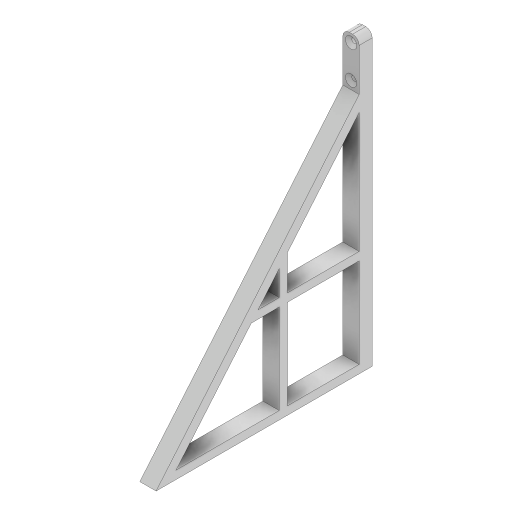
# Autodesk Inventor part: legs
Saved by Autodesk Inventor 2023 (Build 270158000, 158)
## iProperties
Created: 2023-10-18
Part Number: legs
Material: Generic
Document SubType Name: Modeling
Designer: MVeszpremi
Density: 1 g/cm^3
Appearance: Default
Author: MVeszpremi
Autodesk Inventor part; units mm, degrees
ref_plane "YZ Plane" through (0, 0, 0) normal (1, 0, 0) x (0, 1, 0)
ref_plane "XZ Plane" through (0, 0, 0) normal (0, 1, 0) x (-1, 0, 0)
ref_plane "XY Plane" through (0, 0, 0) normal (0, 0, 1) x (1, 0, 0)
sketch "Sketch1" plane through (0, 0, 0) normal (0, 0, 1) x (1, 0, 0)
  line L0 (0, 0) -> (0, 20)
  circle A0 centre (0, 20) radius 1.5
  circle A1 centre (0, 0) radius 1.5
  line L1 (-5, 25) -> (5, 25)
  line L2 (5, 25) -> (5, -5)
  line L3 (5, -5) -> (-5, -5)
  line L4 (-5, -5) -> (-5, 25)
  dimension "d0" = 20
  dimension "d1" = 3
  dimension "d2" = 3
  dimension "d3" = 5
  dimension "d4" = 5
  dimension "d5" = 10
  dimension "d6" = 5
  constraints: 10 end point, 2 centre point, 2 coincident, 2 parallel, 1 horizontal, 1 perpendicular, 1 vertical
  measures "d0" distance of L0.start L0.end
  measures "d1" diameter of A0
  measures "d2" diameter of A1
  measures "d3" distance from line of L1 L0.end
  measures "d4" distance from line of L0.end L4
  measures "d5" distance of L1.start L1.end
  measures "d6" distance from line of L3 L0.start
extrude "Extrusion1" add sketch "Sketch1" along normal blind 8
sketch "Sketch2" plane through (5, -5, 0) normal (1, 0, 0) x (0, 0, -1)
  line L0 (-8, 0) -> (-132.5098, -148.385)
  line L1 (-132.5098, -148.385) -> (-124.5098, -148.385)
  line L2 (-124.5098, -148.385) -> (1.3551, 1.615)
  line L3 (-8, 0) -> (-8, 30) projected
  line L4 (0, 0) -> (0, 30) projected
  line L5 (0, 30) -> (-8, 30) projected
  line L6 (-8, 0) -> (-8, 30) projected
  line L7 (0, 0) -> (-8, 0) projected
  point P0 (0, 5)
  point P1 (0, 0)
  dimension "d9" = 8
  dimension "d10" = 140
  dimension "d11" = 150
  constraints: 6 end point, 1 horizontal, 1 parallel
  measures "d9" distance of L0.end L1.end
  measures "d10" angle of L3 L0
  measures "d11" distance from line of L2.end L1
extrude "Extrusion2" add sketch "Sketch2" against normal up to surface (10 mm away) contours L7 L2 L1 L0
chamfer "Chamfer1" distance 2 angle 45 2 edges at (-1.5, 20, 8) (-1.5, 0, 8)
fillet "Fillet1" radius 4 2 edges at (5, 25, 4) (-5, 25, 4)
sketch "Sketch3" plane through (5, -153.385, 132.5098) normal (1, 0, 0) x (0, 0, -1)
  line L0 (0, 0) -> (8, 0) projected
  line L1 (8, 0) -> (132.5098, 0)
  line L2 (132.5098, 0) -> (132.5098, 5)
  line L3 (132.5098, 5) -> (8, 5)
  line L4 (8, 5) -> (8, 0)
  line L5 (132.5098, 148.6932) -> (124.5098, 148.6932)
  line L6 (124.5098, 148.6932) -> (124.5098, 0)
  line L7 (124.5098, 0) -> (132.5098, 0)
  line L8 (132.5098, 0) -> (132.5098, 148.6932)
  line L9 (124.5098, 148.385) -> (124.5098, 174.385) projected
  line L10 (124.5098, 148.385) -> (0, 0) projected
  line L11 (75.519, 90) -> (80.519, 90)
  line L12 (80.519, 90) -> (80.519, 0)
  line L13 (80.519, 0) -> (75.519, 0)
  line L14 (75.519, 0) -> (75.519, 90)
  line L15 (8, 0) -> (132.5098, 148.385) projected
  line L16 (132.5098, 65) -> (58.346, 65)
  line L17 (58.346, 65) -> (58.346, 60)
  line L18 (58.346, 60) -> (132.5098, 60)
  line L19 (132.5098, 60) -> (132.5098, 65)
  point P0 (132.5098, 153.385)
  point P1 (132.5098, 5)
  point P2 (124.5098, 5)
  point P3 (80.519, 5)
  point P4 (75.519, 5)
  point P5 (80.519, 60)
  point P6 (124.5098, 60)
  point P7 (124.5098, 65)
  point P8 (80.519, 65)
  point P9 (75.519, 60)
  point P10 (75.519, 65)
  dimension "d18" = 5
  dimension "d19" = 5
  dimension "d20" = 90
  dimension "d23" = 5
  dimension "d24" = 55
  constraints: 32 end point, 8 parallel, 6 point on line, 4 horizontal, 4 perpendicular
  measures "d18" distance between parallel lines of L1 L3
  measures "d19" distance of L11.start L11.end
  measures "d20" distance of L11.end L12.end
  measures "d23" distance between parallel lines of L18 L16
  measures "d24" distance between parallel lines of L3 L18
extrude "Extrusion3" add sketch "Sketch3" against normal blind 10 contours L15 L3 L14 L1 | L4 L3 L15 | L11 L12 L15 L14 | L14 L3 L12 L1 | L6 L5 L8 L15 | L15 L12 L16 L14 | L12 L3 L6 L1 | L14 L18 L12 L3 | L17 L16 L15 | L15 L16 L14 L18 | L15 L8 L16 L6 | L16 L12 L18 L14 | L6 L3 L2 L1 | L16 L8 L18 L6 | L6 L18 L12 L16 | L6 L18 L8 L3
body "Solid1"
